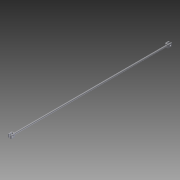
# Autodesk Inventor part: manipulator piston
Saved by Autodesk Inventor 2012 (Build 160160000, 160)
## iProperties
Created: 2013-09-06
Part Number: manipulator piston
Material: Default
Document SubType Name: Modeling
Designer: Bryce
Density: 1 g/cm^3
Author: Bryce
Autodesk Inventor part; units mm, degrees
ref_plane "YZ Plane" through (0, 0, 0) normal (1, 0, 0) x (0, 1, 0)
ref_plane "XZ Plane" through (0, 0, 0) normal (0, 1, 0) x (-1, 0, 0)
ref_plane "XY Plane" through (0, 0, 0) normal (0, 0, 1) x (1, 0, 0)
sketch "Sketch1" plane through (0, 0, 0) normal (0, 0, 1) x (1, 0, 0)
  line L0 (0, 0) -> (12.7, 0)
  line L1 (12.7, 0) -> (12.7, 12.7)
  line L2 (12.7, 12.7) -> (0, 12.7)
  line L3 (0, 12.7) -> (0, 0)
  dimension "d0" = 12.7
  dimension "d1" = 12.7
  constraints: 8 end point, 2 parallel, 1 coincident, 1 horizontal, 1 perpendicular
  measures "d0" distance of L2.end L0.start
  measures "d1" distance of L0.start L0.end
extrude "Extrusion1" add sketch "Sketch1" along normal blind 648.4937
sketch "Sketch2" plane through (12.7, 12.7, 648.4937) normal (0, 1, 0) x (1, 0, 0)
  line L0 (-12.7, 0) -> (0, 0) projected
  line L1 (0, 648.4937) -> (0, 0) projected
  line L2 (0, 648.4937) -> (-12.7, 648.4937) projected
  line L3 (-12.7, 648.4937) -> (-12.7, 0) projected
  line L4 (-12.7, 15.875) -> (-9.525, 15.875)
  line L5 (-9.525, 15.875) -> (-9.525, 632.6187)
  line L6 (-9.525, 632.6187) -> (-12.7, 632.6187)
  line L7 (-12.7, 632.6187) -> (-12.7, 15.875)
  line L8 (0, 632.6187) -> (-3.175, 632.6187)
  line L9 (-3.175, 632.6187) -> (-3.175, 15.875)
  line L10 (-3.175, 15.875) -> (0, 15.875)
  line L11 (0, 15.875) -> (0, 632.6187)
  line L12 (-9.525, 648.4937) -> (-3.175, 648.4937)
  line L13 (-3.175, 648.4937) -> (-3.175, 635.7937)
  line L14 (-3.175, 635.7937) -> (-9.525, 635.7937)
  line L15 (-9.525, 635.7937) -> (-9.525, 648.4937)
  line L16 (-9.525, 0) -> (-3.175, 0)
  line L17 (-3.175, 0) -> (-3.175, 12.7)
  line L18 (-3.175, 12.7) -> (-9.525, 12.7)
  line L19 (-9.525, 12.7) -> (-9.525, 0)
  dimension "d4" = 15.875
  dimension "d5" = 6.35
  dimension "d6" = 15.875
  dimension "d7" = 12.7
  dimension "d8" = 12.7
  constraints: 32 end point, 8 parallel, 7 collinear, 4 horizontal, 4 perpendicular, 4 point on line
  measures "d4" distance between parallel lines of L0 L4
  measures "d5" distance between parallel lines of L9 L5
  measures "d6" distance between parallel lines of L2 L6
  measures "d7" distance between parallel lines of L2 L14
  measures "d8" distance between parallel lines of L0 L18
extrude "Extrusion2" cut sketch "Sketch2" against normal through all contours L19 L18 L17 L0 | L3 L6 L5 L4 | L10 L9 L8 L1 | L2 L13 L14 L15
sketch "Sketch3" plane through (12.7, 0, 648.4937) normal (1, 0, 0) x (0, 0, -1)
  line L0 (15.875, 12.7) -> (0, 12.7) projected
  line L1 (0, 12.7) -> (0, 0) projected
  line L2 (632.6187, 12.7) -> (632.6187, 0) projected
  line L3 (648.4937, 0) -> (632.6187, 0) projected
  line L4 (648.4937, 0) -> (648.4937, 12.7) projected
  line L5 (648.4937, 12.7) -> (632.6187, 12.7) projected
  line L6 (632.6187, 0) -> (15.875, 0) projected
  line L7 (632.6187, 12.7) -> (632.6187, 0) projected
  line L8 (15.875, 12.7) -> (632.6187, 12.7) projected
  line L9 (15.875, 12.7) -> (15.875, 0) projected
  line L10 (15.875, 12.7) -> (632.6187, 12.7)
  line L11 (632.6187, 12.7) -> (632.6187, 9.525)
  line L12 (632.6187, 9.525) -> (15.875, 9.525)
  line L13 (15.875, 9.525) -> (15.875, 12.7)
  line L14 (632.6187, 3.175) -> (15.875, 3.175)
  line L15 (15.875, 3.175) -> (15.875, 0)
  line L16 (15.875, 0) -> (632.6187, 0)
  line L17 (632.6187, 0) -> (632.6187, 3.175)
  circle A0 centre (6.35, 6.35) radius 3.175
  circle A1 centre (642.1437, 6.35) radius 3.175
  point P0 (648.4937, 0)
  dimension "d11" = 6.35
  dimension "d12" = 6.35
  dimension "d13" = 6.35
  dimension "d14" = 6.35
  dimension "d15" = 3.175
  dimension "d16" = 6.35
  dimension "d17" = 6.35
  dimension "d18" = 6.35
  constraints: 16 end point, 4 parallel, 2 centre point, 2 horizontal, 2 perpendicular, 2 point on line
  measures "d11" diameter of A0
  measures "d12" distance from line of L1 A0.centre
  measures "d13" distance from line of L0 A0.centre
  measures "d14" distance between parallel lines of L14 L12
  measures "d15" distance between parallel lines of L12 L8
  measures "d16" diameter of A1
  measures "d17" distance from line of L5 A1.centre
  measures "d18" distance from line of L4 A1.centre
extrude "Extrusion3" cut sketch "Sketch3" against normal through all contours L2 L12 L9 L8 | L2 L6 L9 L14 | A0 | A1
fillet "Fillet1" radius 3.175 4 edges at (9.525, 9.525, 324.2469) (3.175, 9.525, 324.2469) (3.175, 3.175, 324.2469) (9.525, 3.175, 324.2469)
equation "\"d1\" = d0"
equation "\"d13\" = d12"
equation "\"d17\" = d16"
equation "\"d18\" = d17"
body "Solid1"
